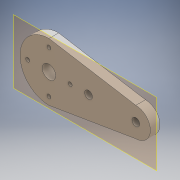
# Autodesk Inventor part: motormount
Saved by Autodesk Inventor 2018 (Build 220112000, 112)
## iProperties
Created: 2017-05-26
Part Number: motormount
Material: Generic
Document SubType Name: Modeling
Designer: Zadeka
Density: 1 g/cm^3
Appearance: Default
Author: Zadeka
Autodesk Inventor part; units mm, degrees
ref_plane "YZ Plane" through (0, 0, 0) normal (1, 0, 0) x (0, 1, 0)
ref_plane "XZ Plane" through (0, 0, 0) normal (0, 1, 0) x (-1, 0, 0)
ref_plane "XY Plane" through (0, 0, 0) normal (0, 0, 1) x (1, 0, 0)
sketch "Sketch1" plane through (0, 0, 0) normal (0, 1, 0) x (-1, 0, 0)
  circle A0 centre (0, 0) radius 22
  line L0 (0, 0) -> (0, -22)
  circle A1 centre (0, -22) radius 1.55
  circle A2 centre (0, -22) radius 3
  circle A3 centre (22, 0) radius 3
  circle A4 centre (22, 0) radius 1.55
  circle A5 centre (0, 22) radius 3
  circle A6 centre (0, 22) radius 1.55
  circle A7 centre (-22, 0) radius 3
  circle A8 centre (-22, 0) radius 1.55
  circle A9 centre (0, 0) radius 30
  line L1 (0, 0) -> (-90, 0)
  circle A10 centre (-90, 0) radius 4
  circle A11 centre (-90, 0) radius 15
  line L2 (0, -30) -> (-90, -15)
  line L3 (0, 30) -> (-90, 15)
  circle A12 centre (0, 0) radius 5
  dimension "d0" = 44
  dimension "d1" = 3.1
  dimension "d2" = 6
  dimension "d5" = 360
  dimension "d7" = 60
  dimension "d8" = 90
  dimension "d9" = 8
  dimension "d10" = 30
  dimension "d11" = 10
  constraints: 12 centre point, 10 coincident, 8 end point, 4 point on circle, 1 horizontal, 1 vertical, 1 vertical alignment, 19 other
  measures "d1" diameter of A1
  measures "d2" diameter of A2
  measures "d7" diameter of A9
  measures "d8" distance of L1.start L1.end
  measures "d9" diameter of A10
  measures "d10" diameter of A11
  measures "d11" diameter of A12
extrude "Extrusion1" add sketch "Sketch1" along normal blind 10 contours A0 A4 | A0 A4 | A4 A0 A3 | A0 A3 A4 | A3 A0 A2 L0 A12 L1 A7 A5 | A9 L3 L2 | A9 L2 A11 L1 | L1 A11 L3 A9 | A5 A0 A6 | A0 A6 A5 | A2 A0 A1 | A0 A1 L0 A2 | A6 A0 | A0 A6 | A1 A0 | A0 L0 A1 | A2 A0 A7 L1 A12 L0 | L0 A1 A0 A2 | A7 L1 A8 A0 | A0 A8 L1 A7 | A0 A1 L0 | A12 L1 L0 | L0 L1 A12 | A8 L1 A0 | A0 L1 A8 | A7 A0 A8 L1 | L1 A8 A0 A7 | L1 A8 A0 | A0 A8 L1 | A11
sketch "Sketch2" plane through (0, 0, 0) normal (0, -1, 0) x (1, 0, 0)
  circle A0 centre (0, 22) radius 1.5
  circle A1 centre (0, -22) radius 1.5
  circle A2 centre (22, 0) radius 1.5
  circle A3 centre (-22, 0) radius 1.5
  circle A4 centre (0, 22) radius 2.05
  circle A5 centre (22, 0) radius 2.05
  circle A6 centre (-22, 0) radius 2.05
  circle A7 centre (0, -22) radius 2.05
  circle A8 centre (-22, 0) radius 2.05
  circle A9 centre (0, 22) radius 2.05
  circle A10 centre (22, 0) radius 2.05
  circle A11 centre (0, -22) radius 2.05
  point P0 (0, 0)
  dimension "d16" = 3
  dimension "d17" = 3
  dimension "d19" = 3
  dimension "d21" = 3
  dimension "d34" = 4.1
  dimension "d35" = 4.1
  dimension "d36" = 4.1
  dimension "d37" = 4.1
  dimension "d38" = 4.1
  dimension "d39" = 4.1
  dimension "d40" = 4.1
  dimension "d41" = 4.1
  constraints: 12 centre point, 8 coincident
  measures "d16" diameter of A0
  measures "d17" diameter of A1
  measures "d19" diameter of A2
  measures "d21" diameter of A3
  measures "d34" diameter of A4
  measures "d35" diameter of A5
  measures "d36" diameter of A6
  measures "d37" diameter of A7
  measures "d38" diameter of A8
  measures "d39" diameter of A9
  measures "d40" diameter of A10
  measures "d41" diameter of A11
extrude "Extrusion2" cut sketch "Sketch2" against normal blind 10 contours A0 | A1 | A2 | A3
sketch "Sketch3" plane through (0, 10, 0) normal (0, 1, 0) x (1, 0, 0)
  circle A0 centre (0, -22) radius 1.5 projected
  line L0 (0, 0) -> (0, -22)
  circle A1 centre (-22, 0) radius 1.5 projected
  line L1 (0, 0) -> (-22, 0)
  circle A2 centre (0, 22) radius 1.5 projected
  line L2 (0, 0) -> (0, 22)
  circle A3 centre (22, 0) radius 1.5 projected
  line L3 (0, 0) -> (22, 0)
  circle A4 centre (0, -22) radius 3
  circle A5 centre (22, 0) radius 3
  circle A6 centre (0, 22) radius 3
  circle A7 centre (-22, 0) radius 3
  dimension "d24" = 6
  dimension "d27" = 360
  constraints: 8 end point, 4 centre point, 2 horizontal, 2 vertical, 1 coincident, 9 other
  measures "d24" diameter of A4
extrude "Extrusion3" cut sketch "Sketch3" against normal blind 3
sketch "Sketch4" plane through (0, 0, 0) normal (0, -1, 0) x (1, 0, 0)
  circle A0 centre (0, 0) radius 5 projected
  circle A1 centre (0, 0) radius 7
  point P0 (0, 0)
  dimension "d31" = 14
  constraints: 1 centre point, 1 coincident
  measures "d31" diameter of A1
extrude "Extrusion4" cut sketch "Sketch4" against normal blind 2.5
ref_plane "Work Plane1" through (0, 0, 0) normal (0, -1, 0) x (1, 0, 0)
sketch "Sketch5" plane through (0, 0, 0) normal (0, -1, 0) x (1, 0, 0)
  circle A0 centre (0, 22) radius 1.5 projected
  circle A1 centre (0, 22) radius 2.05
  circle A2 centre (-22, 0) radius 2.05
  circle A3 centre (0, -22) radius 2.05
  circle A4 centre (22, 0) radius 2.05
  point P0 (0, 0)
  dimension "d43" = 4.1
  dimension "d46" = 360
  constraints: 4 centre point, 1 coincident, 9 other
  measures "d43" diameter of A1
extrude "Extrusion5" cut sketch "Sketch5" against normal blind 10
sketch "Sketch6" plane through (0, 0, 0) normal (0, -1, 0) x (1, 0, 0)
  circle A0 centre (0, 0) radius 7
  constraints: 1 centre point, 1 coincident
extrude "Extrusion6" cut sketch "Sketch6" against normal blind 70.5
sketch "Sketch7" plane through (0, 0, 0) normal (0, -1, 0) x (1, 0, 0)
  circle A0 centre (90, 0) radius 4 projected
  circle A1 centre (41, 0) radius 4
  point P0 (0, 0)
  dimension "d53" = 8
  constraints: 1 centre point
  measures "d53" diameter of A1
extrude "Extrusion7" cut sketch "Sketch7" against normal blind 29.5 contours A1
body "Solid1"
